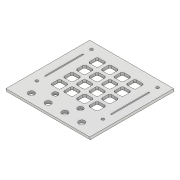
# Autodesk Inventor part: top
Saved by Autodesk Inventor 2017 (Build 210142000, 142)
## iProperties
Created: 2017-03-04
Part Number: top
Material: Acrylic
Document SubType Name: Modeling
Designer: dpgai
Density: 1.188 g/cm^3
Appearance: White
Author: dpgai
Autodesk Inventor part; units mm, degrees
ref_plane "YZ Plane" through (0, 0, 0) normal (1, 0, 0) x (0, 1, 0)
ref_plane "XZ Plane" through (0, 0, 0) normal (0, 1, 0) x (-1, 0, 0)
ref_plane "XY Plane" through (0, 0, 0) normal (0, 0, 1) x (1, 0, 0)
sketch "Sketch1" plane through (0, 0, 0) normal (0, 1, 0) x (-1, 0, 0)
  line L0 (0, 0) -> (100, 0)
  line L1 (100, 0) -> (100, -100)
  line L2 (100, -100) -> (0, -100)
  line L3 (0, -100) -> (0, 0)
  dimension "d0" = 100
  dimension "d1" = 100
  constraints: 8 end point, 2 parallel, 1 horizontal, 1 perpendicular
  measures "d0" distance of L1.end L2.end
  measures "d1" distance of L0.end L1.end
extrude "Extrusion1" add sketch "Sketch1" along normal blind 3.175
sketch "Sketch2" plane through (0, 0, -100) normal (0, 0, -1) x (-1, 0, 0)
  line L0 (0, 0) -> (-0.5598, 3.175)
  line L1 (0, 0) -> (7.4616, 0) construction
  line L2 (0, 0) -> (100, 0) projected
  line L3 (100, 0) -> (99.4402, 3.175)
  line L4 (100, 0) -> (105.9749, 0) construction
  line L5 (100, 3.175) -> (0, 3.175) projected
  line L6 (0, 3.175) -> (-0.5598, 3.175)
  line L7 (0, 3.175) -> (0, 0)
  line L8 (100, 0) -> (100, 3.175)
  dimension "d4" = 100
  dimension "d5" = 100
  constraints: 14 end point, 2 horizontal, 1 collinear, 1 perpendicular, 1 point on line, 1 vertical
  measures "d4" angle of L1 L0
  measures "d5" angle of L4 L3
extrude "Extrusion2" [suppressed]
extrude "Extrusion3" [suppressed]
sketch "Sketch4" plane through (0, 0, 0) normal (0, -1, 0) x (1, 0, 0)
  circle A0 centre (-80, -10.362) radius 3.4985
  line L0 (-76.005, -30.862) -> (-72.5, -30.862)
  line L1 (-78, -32.857) -> (-78, -36.362)
  arc A1 (-76.005, -30.862) -> (-78, -32.857) centre (-76.005, -32.857) ccw
  line L2 (-78, -36.362) -> (-72.5, -36.362) construction
  line L3 (-72.5, -36.362) -> (-72.5, -30.862) construction
  line L4 (-68.995, -30.862) -> (-72.5, -30.862)
  line L5 (-67, -32.857) -> (-67, -36.362)
  arc A2 (-67, -32.857) -> (-68.995, -30.862) centre (-68.995, -32.857) ccw
  line L6 (-76.005, -41.862) -> (-72.5, -41.862)
  line L7 (-78, -39.867) -> (-78, -36.362)
  arc A3 (-78, -39.867) -> (-76.005, -41.862) centre (-76.005, -39.867) ccw
  line L8 (-68.995, -41.862) -> (-72.5, -41.862)
  arc A4 (-68.995, -41.862) -> (-67, -39.867) centre (-68.995, -39.867) ccw
  line L9 (-67, -39.867) -> (-67, -36.362)
  line L10 (-57.5, -36.362) -> (-57.5, -30.862) construction
  line L11 (-52, -32.857) -> (-52, -36.362)
  line L12 (-63, -32.857) -> (-63, -36.362)
  line L13 (-63, -36.362) -> (-57.5, -36.362) construction
  line L14 (-52, -39.867) -> (-52, -36.362)
  arc A5 (-53.995, -41.862) -> (-52, -39.867) centre (-53.995, -39.867) ccw
  line L15 (-53.995, -41.862) -> (-57.5, -41.862)
  line L16 (-61.005, -41.862) -> (-57.5, -41.862)
  line L17 (-63, -39.867) -> (-63, -36.362)
  arc A6 (-63, -39.867) -> (-61.005, -41.862) centre (-61.005, -39.867) ccw
  line L18 (-53.995, -30.862) -> (-57.5, -30.862)
  line L19 (-61.005, -30.862) -> (-57.5, -30.862)
  arc A7 (-61.005, -30.862) -> (-63, -32.857) centre (-61.005, -32.857) ccw
  arc A8 (-52, -32.857) -> (-53.995, -30.862) centre (-53.995, -32.857) ccw
  line L20 (-42.5, -36.362) -> (-42.5, -30.862) construction
  line L21 (-37, -32.857) -> (-37, -36.362)
  line L22 (-48, -32.857) -> (-48, -36.362)
  line L23 (-48, -36.362) -> (-42.5, -36.362) construction
  line L24 (-37, -39.867) -> (-37, -36.362)
  arc A9 (-38.995, -41.862) -> (-37, -39.867) centre (-38.995, -39.867) ccw
  line L25 (-38.995, -41.862) -> (-42.5, -41.862)
  line L26 (-46.005, -41.862) -> (-42.5, -41.862)
  line L27 (-48, -39.867) -> (-48, -36.362)
  arc A10 (-48, -39.867) -> (-46.005, -41.862) centre (-46.005, -39.867) ccw
  line L28 (-38.995, -30.862) -> (-42.5, -30.862)
  line L29 (-46.005, -30.862) -> (-42.5, -30.862)
  arc A11 (-46.005, -30.862) -> (-48, -32.857) centre (-46.005, -32.857) ccw
  arc A12 (-37, -32.857) -> (-38.995, -30.862) centre (-38.995, -32.857) ccw
  line L30 (-27.5, -36.362) -> (-27.5, -30.862) construction
  line L31 (-22, -32.857) -> (-22, -36.362)
  line L32 (-33, -32.857) -> (-33, -36.362)
  line L33 (-33, -36.362) -> (-27.5, -36.362) construction
  line L34 (-22, -39.867) -> (-22, -36.362)
  arc A13 (-23.995, -41.862) -> (-22, -39.867) centre (-23.995, -39.867) ccw
  line L35 (-23.995, -41.862) -> (-27.5, -41.862)
  line L36 (-31.005, -41.862) -> (-27.5, -41.862)
  line L37 (-33, -39.867) -> (-33, -36.362)
  arc A14 (-33, -39.867) -> (-31.005, -41.862) centre (-31.005, -39.867) ccw
  line L38 (-23.995, -30.862) -> (-27.5, -30.862)
  line L39 (-31.005, -30.862) -> (-27.5, -30.862)
  arc A15 (-31.005, -30.862) -> (-33, -32.857) centre (-31.005, -32.857) ccw
  arc A16 (-22, -32.857) -> (-23.995, -30.862) centre (-23.995, -32.857) ccw
  line L40 (-72.5, -51.362) -> (-72.5, -45.862) construction
  line L41 (-67, -47.857) -> (-67, -51.362)
  line L42 (-78, -47.857) -> (-78, -51.362)
  line L43 (-78, -51.362) -> (-72.5, -51.362) construction
  line L44 (-67, -54.867) -> (-67, -51.362)
  arc A17 (-68.995, -56.862) -> (-67, -54.867) centre (-68.995, -54.867) ccw
  line L45 (-68.995, -56.862) -> (-72.5, -56.862)
  line L46 (-76.005, -56.862) -> (-72.5, -56.862)
  line L47 (-78, -54.867) -> (-78, -51.362)
  arc A18 (-78, -54.867) -> (-76.005, -56.862) centre (-76.005, -54.867) ccw
  line L48 (-68.995, -45.862) -> (-72.5, -45.862)
  line L49 (-76.005, -45.862) -> (-72.5, -45.862)
  arc A19 (-76.005, -45.862) -> (-78, -47.857) centre (-76.005, -47.857) ccw
  arc A20 (-67, -47.857) -> (-68.995, -45.862) centre (-68.995, -47.857) ccw
  line L50 (-57.5, -51.362) -> (-57.5, -45.862) construction
  line L51 (-52, -47.857) -> (-52, -51.362)
  line L52 (-63, -47.857) -> (-63, -51.362)
  line L53 (-63, -51.362) -> (-57.5, -51.362) construction
  line L54 (-52, -54.867) -> (-52, -51.362)
  arc A21 (-53.995, -56.862) -> (-52, -54.867) centre (-53.995, -54.867) ccw
  line L55 (-53.995, -56.862) -> (-57.5, -56.862)
  line L56 (-61.005, -56.862) -> (-57.5, -56.862)
  line L57 (-63, -54.867) -> (-63, -51.362)
  arc A22 (-63, -54.867) -> (-61.005, -56.862) centre (-61.005, -54.867) ccw
  line L58 (-53.995, -45.862) -> (-57.5, -45.862)
  line L59 (-61.005, -45.862) -> (-57.5, -45.862)
  arc A23 (-61.005, -45.862) -> (-63, -47.857) centre (-61.005, -47.857) ccw
  arc A24 (-52, -47.857) -> (-53.995, -45.862) centre (-53.995, -47.857) ccw
  line L60 (-42.5, -51.362) -> (-42.5, -45.862) construction
  line L61 (-37, -47.857) -> (-37, -51.362)
  line L62 (-48, -47.857) -> (-48, -51.362)
  line L63 (-48, -51.362) -> (-42.5, -51.362) construction
  line L64 (-37, -54.867) -> (-37, -51.362)
  arc A25 (-38.995, -56.862) -> (-37, -54.867) centre (-38.995, -54.867) ccw
  line L65 (-38.995, -56.862) -> (-42.5, -56.862)
  line L66 (-46.005, -56.862) -> (-42.5, -56.862)
  line L67 (-48, -54.867) -> (-48, -51.362)
  arc A26 (-48, -54.867) -> (-46.005, -56.862) centre (-46.005, -54.867) ccw
  line L68 (-38.995, -45.862) -> (-42.5, -45.862)
  line L69 (-46.005, -45.862) -> (-42.5, -45.862)
  arc A27 (-46.005, -45.862) -> (-48, -47.857) centre (-46.005, -47.857) ccw
  arc A28 (-37, -47.857) -> (-38.995, -45.862) centre (-38.995, -47.857) ccw
  line L70 (-27.5, -51.362) -> (-27.5, -45.862) construction
  line L71 (-22, -47.857) -> (-22, -51.362)
  line L72 (-33, -47.857) -> (-33, -51.362)
  line L73 (-33, -51.362) -> (-27.5, -51.362) construction
  line L74 (-22, -54.867) -> (-22, -51.362)
  arc A29 (-23.995, -56.862) -> (-22, -54.867) centre (-23.995, -54.867) ccw
  line L75 (-23.995, -56.862) -> (-27.5, -56.862)
  line L76 (-31.005, -56.862) -> (-27.5, -56.862)
  line L77 (-33, -54.867) -> (-33, -51.362)
  arc A30 (-33, -54.867) -> (-31.005, -56.862) centre (-31.005, -54.867) ccw
  line L78 (-23.995, -45.862) -> (-27.5, -45.862)
  line L79 (-31.005, -45.862) -> (-27.5, -45.862)
  arc A31 (-31.005, -45.862) -> (-33, -47.857) centre (-31.005, -47.857) ccw
  arc A32 (-22, -47.857) -> (-23.995, -45.862) centre (-23.995, -47.857) ccw
  line L80 (-72.5, -66.362) -> (-72.5, -60.862) construction
  line L81 (-67, -62.857) -> (-67, -66.362)
  line L82 (-78, -62.857) -> (-78, -66.362)
  line L83 (-78, -66.362) -> (-72.5, -66.362) construction
  line L84 (-67, -69.867) -> (-67, -66.362)
  arc A33 (-68.995, -71.862) -> (-67, -69.867) centre (-68.995, -69.867) ccw
  line L85 (-68.995, -71.862) -> (-72.5, -71.862)
  line L86 (-76.005, -71.862) -> (-72.5, -71.862)
  line L87 (-78, -69.867) -> (-78, -66.362)
  arc A34 (-78, -69.867) -> (-76.005, -71.862) centre (-76.005, -69.867) ccw
  line L88 (-68.995, -60.862) -> (-72.5, -60.862)
  line L89 (-76.005, -60.862) -> (-72.5, -60.862)
  arc A35 (-76.005, -60.862) -> (-78, -62.857) centre (-76.005, -62.857) ccw
  arc A36 (-67, -62.857) -> (-68.995, -60.862) centre (-68.995, -62.857) ccw
  line L90 (-57.5, -66.362) -> (-57.5, -60.862) construction
  line L91 (-52, -62.857) -> (-52, -66.362)
  line L92 (-63, -62.857) -> (-63, -66.362)
  line L93 (-63, -66.362) -> (-57.5, -66.362) construction
  line L94 (-52, -69.867) -> (-52, -66.362)
  arc A37 (-53.995, -71.862) -> (-52, -69.867) centre (-53.995, -69.867) ccw
  line L95 (-53.995, -71.862) -> (-57.5, -71.862)
  line L96 (-61.005, -71.862) -> (-57.5, -71.862)
  line L97 (-63, -69.867) -> (-63, -66.362)
  arc A38 (-63, -69.867) -> (-61.005, -71.862) centre (-61.005, -69.867) ccw
  line L98 (-53.995, -60.862) -> (-57.5, -60.862)
  line L99 (-61.005, -60.862) -> (-57.5, -60.862)
  arc A39 (-61.005, -60.862) -> (-63, -62.857) centre (-61.005, -62.857) ccw
  arc A40 (-52, -62.857) -> (-53.995, -60.862) centre (-53.995, -62.857) ccw
  line L100 (-42.5, -66.362) -> (-42.5, -60.862) construction
  line L101 (-37, -62.857) -> (-37, -66.362)
  line L102 (-48, -62.857) -> (-48, -66.362)
  line L103 (-48, -66.362) -> (-42.5, -66.362) construction
  line L104 (-37, -69.867) -> (-37, -66.362)
  arc A41 (-38.995, -71.862) -> (-37, -69.867) centre (-38.995, -69.867) ccw
  line L105 (-38.995, -71.862) -> (-42.5, -71.862)
  line L106 (-46.005, -71.862) -> (-42.5, -71.862)
  line L107 (-48, -69.867) -> (-48, -66.362)
  arc A42 (-48, -69.867) -> (-46.005, -71.862) centre (-46.005, -69.867) ccw
  line L108 (-38.995, -60.862) -> (-42.5, -60.862)
  line L109 (-46.005, -60.862) -> (-42.5, -60.862)
  arc A43 (-46.005, -60.862) -> (-48, -62.857) centre (-46.005, -62.857) ccw
  arc A44 (-37, -62.857) -> (-38.995, -60.862) centre (-38.995, -62.857) ccw
  line L110 (-27.5, -66.362) -> (-27.5, -60.862) construction
  line L111 (-22, -62.857) -> (-22, -66.362)
  line L112 (-33, -62.857) -> (-33, -66.362)
  line L113 (-33, -66.362) -> (-27.5, -66.362) construction
  line L114 (-22, -69.867) -> (-22, -66.362)
  arc A45 (-23.995, -71.862) -> (-22, -69.867) centre (-23.995, -69.867) ccw
  line L115 (-23.995, -71.862) -> (-27.5, -71.862)
  line L116 (-31.005, -71.862) -> (-27.5, -71.862)
  line L117 (-33, -69.867) -> (-33, -66.362)
  arc A46 (-33, -69.867) -> (-31.005, -71.862) centre (-31.005, -69.867) ccw
  line L118 (-23.995, -60.862) -> (-27.5, -60.862)
  line L119 (-31.005, -60.862) -> (-27.5, -60.862)
  arc A47 (-31.005, -60.862) -> (-33, -62.857) centre (-31.005, -62.857) ccw
  arc A48 (-22, -62.857) -> (-23.995, -60.862) centre (-23.995, -62.857) ccw
  line L120 (-72.5, -81.362) -> (-72.5, -75.862) construction
  line L121 (-67, -77.857) -> (-67, -81.362)
  line L122 (-78, -77.857) -> (-78, -81.362)
  line L123 (-78, -81.362) -> (-72.5, -81.362) construction
  line L124 (-67, -84.867) -> (-67, -81.362)
  arc A49 (-68.995, -86.862) -> (-67, -84.867) centre (-68.995, -84.867) ccw
  line L125 (-68.995, -86.862) -> (-72.5, -86.862)
  line L126 (-76.005, -86.862) -> (-72.5, -86.862)
  line L127 (-78, -84.867) -> (-78, -81.362)
  arc A50 (-78, -84.867) -> (-76.005, -86.862) centre (-76.005, -84.867) ccw
  line L128 (-68.995, -75.862) -> (-72.5, -75.862)
  line L129 (-76.005, -75.862) -> (-72.5, -75.862)
  arc A51 (-76.005, -75.862) -> (-78, -77.857) centre (-76.005, -77.857) ccw
  arc A52 (-67, -77.857) -> (-68.995, -75.862) centre (-68.995, -77.857) ccw
  line L130 (-57.5, -81.362) -> (-57.5, -75.862) construction
  line L131 (-52, -77.857) -> (-52, -81.362)
  line L132 (-63, -77.857) -> (-63, -81.362)
  line L133 (-63, -81.362) -> (-57.5, -81.362) construction
  line L134 (-52, -84.867) -> (-52, -81.362)
  arc A53 (-53.995, -86.862) -> (-52, -84.867) centre (-53.995, -84.867) ccw
  line L135 (-53.995, -86.862) -> (-57.5, -86.862)
  line L136 (-61.005, -86.862) -> (-57.5, -86.862)
  line L137 (-63, -84.867) -> (-63, -81.362)
  arc A54 (-63, -84.867) -> (-61.005, -86.862) centre (-61.005, -84.867) ccw
  line L138 (-53.995, -75.862) -> (-57.5, -75.862)
  line L139 (-61.005, -75.862) -> (-57.5, -75.862)
  arc A55 (-61.005, -75.862) -> (-63, -77.857) centre (-61.005, -77.857) ccw
  arc A56 (-52, -77.857) -> (-53.995, -75.862) centre (-53.995, -77.857) ccw
  line L140 (-42.5, -81.362) -> (-42.5, -75.862) construction
  line L141 (-37, -77.857) -> (-37, -81.362)
  line L142 (-48, -77.857) -> (-48, -81.362)
  line L143 (-48, -81.362) -> (-42.5, -81.362) construction
  line L144 (-37, -84.867) -> (-37, -81.362)
  arc A57 (-38.995, -86.862) -> (-37, -84.867) centre (-38.995, -84.867) ccw
  line L145 (-38.995, -86.862) -> (-42.5, -86.862)
  line L146 (-46.005, -86.862) -> (-42.5, -86.862)
  line L147 (-48, -84.867) -> (-48, -81.362)
  arc A58 (-48, -84.867) -> (-46.005, -86.862) centre (-46.005, -84.867) ccw
  line L148 (-38.995, -75.862) -> (-42.5, -75.862)
  line L149 (-46.005, -75.862) -> (-42.5, -75.862)
  arc A59 (-46.005, -75.862) -> (-48, -77.857) centre (-46.005, -77.857) ccw
  arc A60 (-37, -77.857) -> (-38.995, -75.862) centre (-38.995, -77.857) ccw
  line L150 (-27.5, -81.362) -> (-27.5, -75.862) construction
  line L151 (-22, -77.857) -> (-22, -81.362)
  line L152 (-33, -77.857) -> (-33, -81.362)
  line L153 (-33, -81.362) -> (-27.5, -81.362) construction
  line L154 (-22, -84.867) -> (-22, -81.362)
  arc A61 (-23.995, -86.862) -> (-22, -84.867) centre (-23.995, -84.867) ccw
  line L155 (-23.995, -86.862) -> (-27.5, -86.862)
  line L156 (-31.005, -86.862) -> (-27.5, -86.862)
  line L157 (-33, -84.867) -> (-33, -81.362)
  arc A62 (-33, -84.867) -> (-31.005, -86.862) centre (-31.005, -84.867) ccw
  line L158 (-23.995, -75.862) -> (-27.5, -75.862)
  line L159 (-31.005, -75.862) -> (-27.5, -75.862)
  arc A63 (-31.005, -75.862) -> (-33, -77.857) centre (-31.005, -77.857) ccw
  arc A64 (-22, -77.857) -> (-23.995, -75.862) centre (-23.995, -77.857) ccw
  circle A65 centre (-60, -10.362) radius 3.4985
  circle A66 centre (-40, -10.362) radius 3.4985
  circle A67 centre (-20, -10.362) radius 3.4985
  circle A68 centre (-65, -23.862) radius 3.15
  line L160 (-52, -35.3195) -> (-48, -35.3195) construction
  line L161 (-50, -35.3195) -> (-50, -12.8531) construction
  circle A69 centre (-35, -23.862) radius 3.15
  line L162 (-11.225, -36.112) -> (-9.975, -36.112)
  line L163 (-9.975, -36.112) -> (-9.975, -81.612)
  line L164 (-9.975, -81.612) -> (-11.225, -81.612)
  line L165 (-11.225, -81.612) -> (-11.225, -36.112)
  circle A70 centre (-10.6, -26.287) radius 1.7
  circle A71 centre (-10.6, -91.437) radius 1.7
  line L166 (-88.775, -36.112) -> (-90.025, -36.112)
  line L167 (-90.025, -36.112) -> (-90.025, -81.612)
  line L168 (-90.025, -81.612) -> (-88.775, -81.612)
  line L169 (-88.775, -81.612) -> (-88.775, -36.112)
  circle A72 centre (-89.4, -26.287) radius 1.7
  circle A73 centre (-89.4, -91.437) radius 1.7
  line L170 (-100, 0) -> (-100, -100) projected
  line L171 (0, -100) -> (0, 0) projected
  dimension "d13" = 6.997
  dimension "d19" = 3.99
  dimension "d24" = 5.5
  dimension "d27" = 15
  dimension "d30" = 15
  dimension "d34" = 20.5
  dimension "d37" = 20
  dimension "d42" = 6.3
  dimension "d43" = 15
  dimension "d44" = 6.3
  dimension "d45" = 15
  dimension "d46" = 7
  dimension "d47" = 7
  dimension "d48" = 1.25
  dimension "d49" = 45.5
  dimension "d52" = 3.4
  dimension "d53" = 9.825
  dimension "d54" = 3.4
  dimension "d55" = 9.825
  dimension "d65" = 20
  dimension "d66" = 20
  constraints: 340 end point, 128 point on circle, 74 centre point, 17 symmetric about line, 5 horizontal, 4 perpendicular, 2 collinear, 2 parallel, 2 point on line, 2 tangent, 2 vertical, 1 midpoint, 474 other
  measures "d13" diameter of A0
  measures "d19" diameter of A1
  measures "d24" distance between parallel lines of L2 L0
  measures "d27" distance of L2.end L10.start
  measures "d30" distance of L2.end L40.start
  measures "d34" distance from line of L4 A0.centre
  measures "d37" distance of A0.centre A65.centre
  measures "d42" diameter of A68
  measures "d43" horizontal distance of L161.start A68.centre
  measures "d44" diameter of A69
  measures "d45" distance from line of L161 A69.centre
  measures "d46" distance from line of L19 A68.centre
  measures "d47" distance from line of L39 A69.centre
  measures "d48" distance of L163.end L164.end
  measures "d49" distance of L162.end L163.end
  measures "d52" diameter of A70
  measures "d53" distance from line of L162 A70.centre
  measures "d54" diameter of A71
  measures "d55" distance from line of L164 A71.centre
  measures "d65" distance from line of L170 A0.centre
  measures "d66" distance from line of L171 A67.centre
extrude "Extrusion5" cut sketch "Sketch4" against normal through all
sketch "Sketch5" plane through (-100, 0, -100) normal (-1, 0, 0) x (0, 0, 1)
  line L0 (0, 3.175) -> (-0.5598, 0)
  line L1 (0, 3.175) -> (6.0716, 3.175) construction
  line L2 (0, 0) -> (0, 3.175) projected
  line L3 (0, 0) -> (-0.5598, 0)
  line L4 (100, 0) -> (100, 3.175) projected
  line L5 (100, 0) -> (100, 3.175) projected
  line L6 (100, 3.175) -> (99.4402, 0)
  line L7 (100, 3.175) -> (107.5546, 3.175) construction
  line L8 (100, 0) -> (99.4402, 0)
  line L9 (100, 0) -> (0, 0) projected
  dimension "d58" = 100
  dimension "d60" = 100
  constraints: 12 end point, 3 horizontal, 1 point on line
  measures "d58" angle of L0 L1
  measures "d60" angle of L6 L7
extrude "Extrusion6" cut sketch "Sketch5" against normal blind 100 contours L6 L4 L8
extrude "Extrusion7" add sketch "Sketch5" against normal blind 100 contours L2 L3 L0
body "Solid1"
